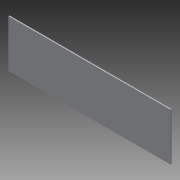
# Autodesk Inventor part: blacha2
Saved by Autodesk Inventor 2014 (Build 180170000, 170)
## iProperties
Created: 2013-08-20
Part Number: blacha2
Material: Aluminium 6061
Document SubType Name: Konstrukcja blachowa
Designer: Kisieel
Density: 1 g/cm^3
Flat Pattern Width: 8.8 cm
Flat Pattern Length: 30 cm
Flat Pattern Area: 264 cm^2
Sheet Metal Rule: Domyślny
Sheet Metal Width: 88,000 mm
Sheet Metal Length: 300,000 mm
Sheet Metal Area: 26400,000 mm^2
Appearance: Aluminium — płaski
Author: Kisieel
Autodesk Inventor part; units mm, degrees
ref_plane "YZ Plane" through (0, 0, 0) normal (1, 0, 0) x (0, 1, 0)
ref_plane "XZ Plane" through (0, 0, 0) normal (0, 1, 0) x (-1, 0, 0)
ref_plane "XY Plane" through (0, 0, 0) normal (0, 0, 1) x (1, 0, 0)
sketch "Szkic1" plane through (0, 0, 0) normal (0, 1, 0) x (-1, 0, 0)
  line L0 (0, 0) -> (300, 0)
  line L1 (300, 0) -> (300, 88)
  line L2 (300, 88) -> (0, 88)
  line L3 (0, 88) -> (0, 0)
  dimension "d0" = 300
  dimension "d2" = 88
  constraints: 8 end point, 2 parallel, 1 horizontal, 1 perpendicular
  measures "d0" distance of L1.end L2.end
  measures "d2" distance of L2.end L0.start
extrude "Wyciągnięcie proste1" add sketch "Szkic1" along normal blind 4
equation "\"PromieńGięcia\" = Grubość"
equation "\"SzerokośćGięciaPodcięcia\" = Grubość"
equation "\"GłębokośćGięciaPodcięcia\" = 0.5 * Grubość"
equation "\"RozmiarPodcięciaNarożnika\" = 4 * Grubość"
equation "\"MinimalnaPozostałość\" = 2 * Grubość"
equation "\"PromieńPrzejścia\" = PromieńGięcia"
equation "\"Rozmiar_promienia_Jacobiego\" = Grubość"
equation "\"Wielk_odstępu\" = Grubość"
equation "\"Grubość\" = 4"
